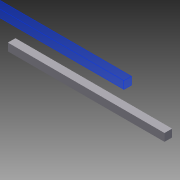
# Autodesk Inventor part: SupportBar
Saved by Autodesk Inventor 2012 (Build 160160000, 160)
## iProperties
Created: 2012-04-10
Part Number: SupportBar
Material: Aluminum-6061
Document SubType Name: Modeling
Designer: admin
Density: 2.71 g/cm^3
Mass: 46.0066 g
Surface Area: 80.0007 cm^2
Volume: 16.9766 cm^3
Author: admin
Autodesk Inventor part; units mm, degrees
ref_plane "YZ Plane" through (0, 0, 0) normal (1, 0, 0) x (0, 1, 0)
ref_plane "XZ Plane" through (0, 0, 0) normal (0, 1, 0) x (-1, 0, 0)
ref_plane "XY Plane" through (0, 0, 0) normal (0, 0, 1) x (1, 0, 0)
sketch "Sketch1" plane through (0, 0, 0) normal (0, 0, 1) x (1, 0, 0)
  line L0 (0, 0) -> (195.58, 0)
  line L1 (195.58, 0) -> (195.58, 9.525)
  line L2 (195.58, 9.525) -> (0, 9.525)
  line L3 (0, 9.525) -> (0, 0)
  dimension "d0" = 9.525
  dimension "d1" = 195.58
  constraints: 8 end point, 2 parallel, 1 horizontal, 1 perpendicular
  measures "d0" distance between parallel lines of L0 L2
  measures "d1" distance between parallel lines of L1 L3
extrude "Extrusion1" add sketch "Sketch1" along normal blind 9.525
sketch "Sketch2" plane through (0, 9.525, 0) normal (0, 1, 0) x (1, 0, 0)
  line L0 (195.58, 0) -> (0, 0) projected
  line L1 (9.525, 0) -> (9.525, -9.525) projected
  line L2 (73.66, -9.525) -> (73.66, 0) projected
  line L3 (83.185, 0) -> (83.185, -9.525) projected
  line L4 (112.395, 0) -> (112.395, -9.525) projected
  line L5 (121.92, -9.525) -> (121.92, 0) projected
  line L6 (186.055, 0) -> (186.055, -9.525) projected
  point P0 (4.7625, -4.7625)
  point P1 (78.4225, -4.7625)
  point P2 (117.1575, -4.7625)
  point P3 (190.8175, -4.7625)
  dimension "d4" = 4.7625
  dimension "d5" = 4.7625
  dimension "d6" = 4.7625
  dimension "d7" = 4.7625
  dimension "d8" = 4.7625
  dimension "d9" = 4.7625
  dimension "d10" = 4.7625
  dimension "d11" = 4.7625
  measures "d4" distance from line of L0 point (4.763, -4.763)
  measures "d5" distance from line of L2 point (78.423, -4.763)
  measures "d6" distance from line of L0 point (78.423, -4.763)
  measures "d7" distance from line of L4 point (117.157, -4.763)
  measures "d8" distance from line of L0 point (117.157, -4.763)
  measures "d9" distance from line of L0 point (190.818, -4.763)
  measures "d10" distance from line of L6 point (190.818, -4.763)
  measures "d11" distance from line of L1 point (4.763, -4.763)
hole "Hole1" at (4.7625, 9.525, 4.7625) at (78.4225, 9.525, 4.7625) at (117.1575, 9.525, 4.7625) at (190.8175, 9.525, 4.7625) direction (0, -1, 0) diameter 4.4958 end through all countersink diameter 8.4328 countersink angle 82 clearance for "Flat Head Machine Screw (82)" size "#8" standard "Ansi Unified Screw Threads"
body "Solid1"
